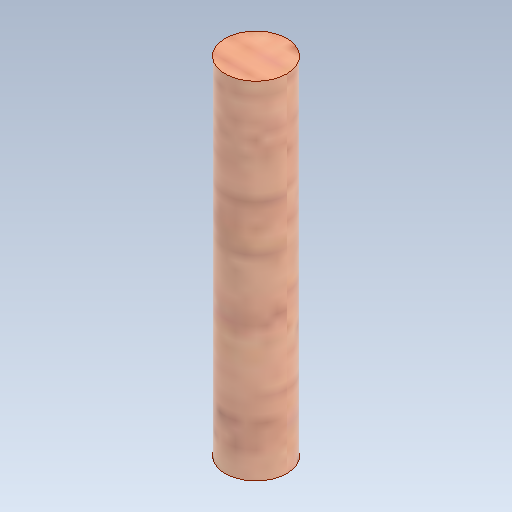
# Autodesk Inventor part: Tarugos
Saved by Autodesk Inventor 2020.3 (Build 243373000, 373)
## iProperties
Created: 2020-10-27
Part Number: Tarugos
Material: Madera (roble)
Document SubType Name: Modeling
Designer: codig
Density: 0.76 g/cm^3
Appearance: Roble blanco - Natural brillo medio
Author: codig
Autodesk Inventor part; units mm, degrees
ref_plane "YZ Plane" through (0, 0, 0) normal (1, 0, 0) x (0, 1, 0)
ref_plane "XZ Plane" through (0, 0, 0) normal (0, 1, 0) x (-1, 0, 0)
ref_plane "XY Plane" through (0, 0, 0) normal (0, 0, 1) x (1, 0, 0)
sketch "Boceto1" plane through (0, 0, 0) normal (0, 1, 0) x (-1, 0, 0)
  circle A0 centre (0, 0) radius 4
  dimension "d1" = 45
  constraints: 1 centre point, 1 coincident
extrude "Extrusión1" add sketch "Boceto1" along normal blind 45
